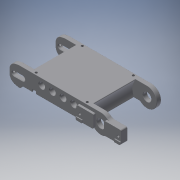
# Autodesk Inventor part: J007811
Saved by Autodesk Inventor 2018.3 (Build 223284000, 284)
## iProperties
Created: 2014-06-24
Material: VERO BLACK
Vendor: HHMI: JRC - ID&F
Document SubType Name: Modeling
Designer: ARNOLDJ
Density: 1.17 g/cm^3
Description: NRB MAIN BODY INSERTS
Mass: 114.449 g
Surface Area: 315.275 cm^2
Volume: 97.8198 cm^3
Appearance: Default
Project: COMMON
Part Number: J007811
RuleStatus: InUse
AfterDocSave0: file://Part Number Cleaner
LAB/DEPT: COMMON
REQUESTING SCIENTIST: COMMON
SURFACE ROUGHNESS: N/A
DESIGN DEPARTMENT: HHMI: JRC - ID&F
SPECIAL FINISH: NONE
ALTERED ITEM PART NUMBER: N/A
ALTERED ITEM VENDOR: N/A
ALTERED ITEM DESCRIPTION: N/A
Revision Number: 0
Autodesk Inventor part; units mm, degrees
sketch "Sketch1" plane through (0, 0, 0) normal (0, 0, 1) x (1, 0, 0)
  circle A0 centre (0, 0) radius 2.286
  circle A1 centre (98.552, 0) radius 4.7752
  line L0 (-5.7162, 13.208) -> (130.4794, 13.208) construction
  line L1 (0, 11.708) -> (98.552, 11.708)
  arc A2 (90.2495, -8.255) -> (98.552, 11.708) centre (98.552, 0) ccw
  line L2 (5.358, -8.255) -> (90.2495, -8.255)
  line L3 (0, 0) -> (0, -11.708) construction
  line L4 (0, -11.708) -> (-26.2981, -11.708) construction
  circle A3 centre (98.552, 0) radius 13.208 construction
  arc A4 (-3.81, 11.708) -> (-3.81, -11.708) centre (-3.81, 0) ccw
  line L5 (-3.81, -11.708) -> (1.905, -11.708)
  line L6 (-3.81, 11.708) -> (0, 11.708)
  circle A5 centre (98.552, 0) radius 11.708 construction
  line L7 (1.905, -11.708) -> (5.358, -8.255)
  circle A6 centre (-3.81, 0) radius 17.399 construction
  line L8 (-10.795, 9.3961) -> (-10.795, -9.3961)
  line L9 (0, 11.708) -> (-10.795, 9.3961)
  line L10 (-10.795, -9.3961) -> (0, -11.708)
  dimension "d233" = 23.416
  dimension "BRG_CLEAR" = 4.572
  dimension "d1" = 9.5504
  dimension "AXEL_CENTER" = 98.552
  dimension "TOP_CHAIN" = 13.208
  dimension "BELT_THICKNESS" = 1.5
  dimension "d111" = 3.81
  dimension "d226" = 11.708
  dimension "d232" = 8.255
  dimension "d235" = 135
  dimension "d236" = 1.905
  dimension "d237" = 26.416
  dimension "d238" = 34.798
  dimension "d335" = 10.795
  constraints: 22 end point, 6 centre point, 6 coincident, 6 point on circle, 5 horizontal, 4 tangent, 2 point on line, 2 vertical, 1 equal radius, 1 horizontal alignment, 1 parallel, 3 other
  measures "BRG_CLEAR" diameter of A0
  measures "d1" diameter of A1
  measures "AXEL_CENTER" distance of A1.centre point (0, 0)
  measures "TOP_CHAIN" distance from line of L0 point (0, 0)
  measures "BELT_THICKNESS" distance between parallel lines of L1 L0
  measures "d111" distance of point (0, 0) A4.centre
  measures "d226" distance from line of L1 point (0, 0)
  measures "d232" distance from line of L2 A1.centre
  measures "d235" angle of L2 L7
  measures "d236" horizontal distance of point (0, 0) L5.end
  measures "d237" diameter of A3
  measures "d238" diameter of A6
  measures "d335" distance from line of point (0, 0) L8
extrude "Extrusion1" add sketch "Sketch1" along normal mid plane 60.198 contours L1 A2 L2 L7 L5 L10 L8 L9
ref_plane "Work Plane1" through (0, 0, 6.5) normal (0, 0, 1) x (1, 0, 0)
sketch "Sketch2" plane through (0, 0, 6.5) normal (0, 0, 1) x (1, 0, 0)
  circle A0 centre (98.552, 0) radius 4.7752 projected
  circle A1 centre (0, 0) radius 2.286 projected
  line L0 (98.552, 11.708) -> (0, 11.708) projected
  arc A2 (90.2495, -8.255) -> (98.552, 11.708) centre (98.552, 0) ccw projected
  line L1 (5.358, -8.255) -> (90.2495, -8.255) projected
  line L2 (0, -11.708) -> (1.905, -11.708) projected
  line L3 (1.905, -11.708) -> (5.358, -8.255) projected
  line L4 (-10.795, 9.3961) -> (-10.795, -9.3961) projected
  line L5 (0, 11.708) -> (-10.795, 9.3961) projected
  line L6 (-10.795, -9.3961) -> (0, -11.708) projected
sketch "Sketch14" plane through (0, 0, 0) normal (0, 0, 1) x (1, 0, 0)
  point P0 (0, 0)
sketch "Sketch15" plane through (0, 0, 0) normal (0, 0, 1) x (1, 0, 0)
  line L0 (0, 11.708) -> (98.552, 11.708) projected
  circle A0 centre (98.552, 0) radius 4.7752 projected
  line L1 (90.2495, -8.255) -> (5.358, -8.255) projected
  circle A1 centre (98.552, 0) radius 17.4625
  circle A2 centre (0, 0) radius 2.286 projected
  circle A3 centre (0, 0) radius 17.4625
  circle A4 centre (-3.81, 0) radius 17.4625
  line L2 (-3.81, 17.4625) -> (0, 17.4625)
  dimension "d241" = 34.925
  dimension "d242" = 34.925
  dimension "d239" = 34.925
  constraints: 2 coincident, 2 end point, 2 horizontal, 2 vertical alignment, 1 centre point, 4 other
  measures "d239" diameter of A1
extrude "Extrusion6" cut sketch "Sketch15" along normal mid plane 50.038 contours A4 A3 L0 | L0 A3 L1 A4 | A4 A3 | A3 A4 | A1 | L1 A3 A4
fillet "Fillet13" radius 0.635 4 edges at (85.5959, 11.708, 0) (83.1639, -8.255, 0) (12.9561, 11.708, 0) (15.3881, -8.255, 0)
sketch "Sketch17" plane through (0, 0, 0) normal (0, 1, 0) x (-1, 0, 0)
  line L0 (-151.1165, 0) -> (65.8274, 0) projected
  line L1 (-118.2232, 10.8) -> (28.7239, 10.8) construction
  line L2 (-120.1245, -10.8) -> (34.8354, -10.8) construction
  point P0 (0, 0)
  dimension "d89" = 10.8
  dimension "d90" = 10.8
  constraints: 4 end point, 2 horizontal
  measures "d89" distance between parallel lines of L0 L1
  measures "d90" distance between parallel lines of L0 L2
sketch "Sketch18" plane through (0, 0, 0) normal (1, 0, 0) x (0, 1, 0)
  line L0 (-19.3771, 6.985) -> (16.5156, 6.985) construction
  line L1 (-20.38, -6.985) -> (18.235, -6.985) construction
  line L2 (-28.1031, 0) -> (25.958, 0) construction
  line L3 (0, 35.0266) -> (0, -35.0266) construction
  line L4 (11.708, 7.62) -> (11.073, 7.62)
  line L5 (11.073, 7.62) -> (11.073, 6.35)
  line L6 (11.073, 6.35) -> (11.708, 6.35)
  line L7 (11.708, 6.35) -> (11.708, 7.62)
  line L8 (11.708, -6.35) -> (11.073, -6.35)
  line L9 (11.073, -6.35) -> (11.073, -7.62)
  line L10 (11.073, -7.62) -> (11.708, -7.62)
  line L11 (11.708, -7.62) -> (11.708, -6.35)
  line L12 (11.708, 25.019) -> (11.708, -25.019) projected
  point P0 (0, 0)
  dimension "d94" = 0.635
  dimension "d243" = 0
  dimension "d244" = 0
  dimension "d367" = 12.7
  dimension "d368" = 1.27
  constraints: 20 end point, 4 horizontal, 4 parallel, 2 equal length, 2 perpendicular, 2 other
  measures "d94" distance of L4.start L4.end
  measures "d243" distance between parallel lines of L11 L12
  measures "d244" distance between parallel lines of L7 L12
  measures "d367" distance between parallel lines of L8 L6
  measures "d368" distance of L4.end L5.end
extrude "Extrusion8" [suppressed]
sketch "Sketch19" plane through (0, 0, 0) normal (0, 0, 1) x (1, 0, 0)
  line L0 (0, 0) -> (0, 6.4329) construction
  circle A0 centre (-5.08, 0) radius 2.413
  circle A1 centre (5.08, 0) radius 2.413
  line L1 (5.08, 0) -> (5.08, 2.413) construction
  line L2 (-5.08, 0) -> (-5.08, 2.413) construction
  line L3 (-5.08, 0) -> (-5.08, -2.413) construction
  line L4 (5.08, 0) -> (5.08, -2.413) construction
  line L5 (-5.08, 2.413) -> (5.08, 2.413)
  line L6 (-5.08, -2.413) -> (5.08, -2.413)
  arc A2 (0, 8.9) -> (3.6068, -8.1364) centre (0, 0) ccw construction
  dimension "d105" = 4.826
  dimension "d106" = 5.08
  dimension "d107" = 10.16
  constraints: 14 end point, 5 vertical, 4 point on circle, 4 tangent, 2 centre point, 2 horizontal, 1 equal radius
  measures "d105" diameter of A0
  measures "d106" distance of L2.start L0.start
  measures "d107" distance of L1.start L2.start
extrude "Extrusion9" cut sketch "Sketch19" along normal mid plane 88.9
mirror "Mirror4" about plane through (0, 0, 0) normal (0, 0, 1)
ref_plane "Work Plane3" through (0, 0, -28.5496) normal (0, 0, 1) x (1, 0, 0)
ref_plane "Work Plane5" through (-19.05, 0, 0) normal (1, 0, 0) x (0, 1, 0)
sketch "Sketch31" plane through (-19.05, 0, 0) normal (1, 0, 0) x (0, 1, 0)
  line L0 (9.3961, -30.099) -> (-9.3961, -30.099) projected
  line L1 (-9.3961, 30.099) -> (9.3961, 30.099) projected
  line L2 (-9.3961, -25.019) -> (9.3961, -25.019) projected
  line L3 (9.3961, 25.019) -> (-9.3961, 25.019) projected
  line L4 (0, 42.1386) -> (0, -42.1386) projected
  point P0 (0, 0)
  point P1 (0, -27.559)
  point P2 (0, 27.559)
  dimension "d338" = 5.08
  dimension "d339" = 2.54
  dimension "d403" = 0
  dimension "d404" = 2.54
  constraints: 1 vertical alignment
  measures "d338" distance between parallel lines of L0 L2
  measures "d339" distance from line of point (0, -27.559) L0
  measures "d403" distance from line of L4 point (0, -27.559)
  measures "d404" distance from line of point (0, 27.559) L3
hole "Hole6" at (-19.05, 0, -27.559) at (-19.05, 0, 27.559) direction (1, 0, 0) diameter 2.3622 depth 19.05 tip angle 118
ref_plane "Work Plane6" through (0, 0, 12.5095) normal (0, 0, 1) x (1, 0, 0)
ref_plane "Work Plane7" through (0, 0, 25.019) normal (0, 0, 1) x (1, 0, 0)
hole "Hole7" at (98.552, 0, 25.019) direction (0, 0, 1) diameter 9.5758 depth 25.4 tip angle 118
ref_plane "Work Plane9-Motor Drive Plane" through (135.1026, 0, 0) normal (1, 0, 0) x (0, 1, 0)
fillet "Fillet21" radius 2.54 5 edges at (1.905, -11.708, 27.559) (5.358, -8.255, 27.559) (1.905, -11.708, -27.559) (5.358, -8.255, -27.559) (90.2495, -8.255, -27.559)
fillet "Fillet22" radius 8.89 6 edges at (-10.795, 9.3961, -27.559) (-10.795, -9.3961, 27.559) (-10.795, -9.3961, -27.559) (-10.795, 9.3961, 27.559) (0, 11.708, -27.559) (0, 11.708, 27.559)
sketch "Sketch40" plane through (0, 0, 25.019) normal (0, 0, 1) x (1, 0, 0)
  circle A0 centre (98.552, 0) radius 4.7879 projected
  line L0 (0.9413, 11.708) -> (98.552, 11.708) projected
  arc A1 (90.2495, -8.255) -> (98.552, 11.708) centre (98.552, 0) ccw projected
  line L1 (90.2495, -8.255) -> (6.4101, -8.255) projected
  line L2 (92.202, -7.62) -> (71.882, -7.62)
  line L3 (71.882, -7.62) -> (71.882, 7.62)
  line L4 (71.882, 7.62) -> (92.202, 7.62)
  line L5 (92.202, 7.62) -> (92.202, -7.62)
  line L6 (92.202, -7.62) -> (71.882, 7.62) construction
  line L7 (71.882, -7.62) -> (92.202, 7.62) construction
  line L8 (104.902, -7.62) -> (125.222, -7.62)
  line L9 (125.222, -7.62) -> (125.222, 7.62)
  line L10 (125.222, 7.62) -> (104.902, 7.62)
  line L11 (104.902, 7.62) -> (104.902, -7.62)
  line L12 (104.902, -7.62) -> (125.222, 7.62) construction
  line L13 (125.222, -7.62) -> (104.902, 7.62) construction
  point P0 (0, 0)
  point P1 (82.042, 0)
  point P2 (115.062, 0)
  point P3 (82.042, 0)
  point P4 (115.062, 0)
  dimension "d343" = 6.35
  dimension "d344" = 6.35
  dimension "d345" = 26.67
  dimension "d346" = 26.67
  dimension "d347" = 15.24
  dimension "d348" = 15.24
  constraints: 24 end point, 6 midpoint, 4 parallel, 2 horizontal, 2 horizontal alignment, 2 perpendicular
  measures "d343" distance from line of L5 A0.centre
  measures "d344" distance from line of L11 A0.centre
  measures "d345" distance from line of A1.centre L3
  measures "d346" distance from line of L9 A0.centre
  measures "d347" distance of L2.end L3.end
  measures "d348" distance of L8.end L9.end
extrude "Extrusion22" add sketch "Sketch40" along normal blind 7.62 contours L8 L11 L10 A1 | A1 L10 L9 L8 | L2 L3 L4 L5
sketch "Sketch41" plane through (0, 0, 32.639) normal (0, 0, 1) x (1, 0, 0)
  circle A0 centre (98.552, 0) radius 4.7879 projected
  circle A1 centre (98.552, 0) radius 23 construction
  line L0 (71.882, -7.62) -> (79.502, -7.62)
  line L1 (79.502, -7.62) -> (79.502, -4.2418)
  line L2 (79.502, -4.2418) -> (71.882, -4.2418)
  line L3 (71.882, -4.2418) -> (71.882, -7.62)
  line L4 (125.222, -7.62) -> (117.602, -7.62)
  line L5 (117.602, -7.62) -> (117.602, -4.2418)
  line L6 (117.602, -4.2418) -> (125.222, -4.2418)
  line L7 (125.222, -4.2418) -> (125.222, -7.62)
  point P0 (0, 0)
  point P1 (75.552, 0)
  point P2 (121.552, 0)
  dimension "d351" = 46
  dimension "d359" = 7.62
  dimension "d360" = 7.62
  dimension "d361" = 4.2418
  constraints: 16 end point, 4 parallel, 2 horizontal, 2 perpendicular, 2 point on circle, 1 centre point, 1 coincident, 1 horizontal alignment, 1 point on line
  measures "d351" diameter of A1
  measures "d359" distance of L1.end L2.end
  measures "d360" distance of L5.end L6.end
  measures "d361" distance from line of L2 A1.start
hole "Hole8" at (75.552, 0, 32.639) at (121.552, 0, 32.639) direction (0, 0, -1) diameter 2.8956 depth 20.32 tip angle 118 clearance for "Socket Head Cap Screw" size "M2.5" standard "Ansi Metric M Profile"
ref_plane "Work Plane10" through (0, 0, 42.164) normal (0, 0, 1) x (1, 0, 0)
sketch "Sketch5" plane through (0, 0, 42.164) normal (0, 0, 1) x (1, 0, 0)
  circle A0 centre (97.79, 0) radius 4.7879
  circle A1 centre (-9.5263, 0.1013) radius 2.286
  line L0 (-75.7985, 4.088) -> (143.5735, 4.088)
  line L1 (0, 18.1055) -> (0, -20.875) projected
  line L2 (0.9413, 11.708) -> (98.552, 11.708) projected
  point P0 (27.94, 4.088)
  point P1 (53.34, 4.088)
  point P2 (40.64, 4.088)
  point P3 (66.04, 4.088)
  dimension "d33" = 25.4
  dimension "d34" = 12.7
  dimension "d405" = 40.64
  dimension "d406" = 7.62
  dimension "d407" = 3.9867
  dimension "d408" = 12.7
  constraints: 4 point on line, 2 centre point, 2 end point, 2 horizontal alignment
  measures "d33" distance of point (53.34, 4.088) point (27.94, 4.088)
  measures "d34" distance of point (53.34, 4.088) point (40.64, 4.088)
  measures "d405" distance from line of point (40.64, 4.088) L1
  measures "d406" distance from line of point (27.94, 4.088) L2
  measures "d407" vertical distance of point (27.94, 4.088) A1.centre
  measures "d408" distance of point (66.04, 4.088) point (53.34, 4.088)
hole "Hole2" at (27.94, 4.088, 42.164) at (53.34, 4.088, 42.164) at (40.64, 4.088, 42.164) at (66.04, 4.088, 42.164) direction (0, 0, -1) diameter 6.731 end through all
extrude "Extrusion23" add sketch "Sketch41" along normal blind 1.016 contours L3 L2 L1 L0 | L4 L5 L6 L7
fillet "Fillet23" radius 1.524 8 edges at (71.882, 7.62, 31.369) (92.202, 7.62, 31.369) (92.202, -7.62, 31.369) (104.902, 7.62, 31.369) (125.222, 7.62, 28.829) (125.222, -7.62, 29.337) (104.902, -7.62, 31.369) (71.882, -7.62, 31.877)
chamfer "Chamfer12" distance 0.381 angle 45 4 edges at (93.7768, 0, -30.099) (98.552, -4.7879, 30.099) (98.552, -4.7879, 25.019) (93.7768, 0, -25.019)
fillet "Fillet24" radius 6.35 2 edges at (107.4409, 7.62, 27.559) (107.4409, -7.62, 27.559)
fillet "Fillet25" radius 0.635 6 edges at (79.502, -4.2418, 33.147) (79.502, -7.62, 33.147) (71.882, -4.2418, 33.147) (117.602, -4.2418, 33.147) (125.222, -4.2418, 33.147) (117.602, -7.62, 33.147)
sketch "Sketch46" plane through (0, 0, 0) normal (0, 0, 1) x (1, 0, 0)
  circle A0 centre (27.94, 4.088) radius 3.3655 projected
  line L0 (22.352, 9.676) -> (33.528, 9.676)
  line L1 (33.528, 9.676) -> (33.528, -1.5)
  line L2 (33.528, -1.5) -> (22.352, -1.5)
  line L3 (22.352, -1.5) -> (22.352, 9.676)
  line L4 (22.352, 9.676) -> (33.528, -1.5) construction
  line L5 (33.528, 9.676) -> (22.352, -1.5) construction
  point P0 (0, 0)
  dimension "d409" = 11.176
  dimension "d410" = 11.176
  constraints: 12 end point, 2 midpoint, 2 parallel, 1 horizontal, 1 perpendicular
  measures "d409" distance of L1.end L2.end
  measures "d410" distance of L0.end L1.end
extrude "Extrusion26" cut sketch "Sketch46" along normal mid plane 48.26 contours A0 | L0 L1 L2 L3
pattern_linear "Rectangular Pattern2" count 4 spacing 12.7 along (1, 0, 0) of "Extrusion26"
sketch "Sketch42" plane through (90.2495, -8.255, 25.019) normal (0, -1, 0) x (1, 0, 0)
  line L0 (-90.2495, 21.3868) -> (-90.2495, -67.8688) projected
  line L1 (-157.0964, -25.019) -> (66.984, -25.019) projected
  line L2 (-13.0335, -42.799) -> (-68.9135, -42.799)
  line L3 (-68.9135, -42.799) -> (-68.9135, -7.239)
  line L4 (-68.9135, -7.239) -> (-13.0335, -7.239)
  line L5 (-13.0335, -7.239) -> (-13.0335, -42.799)
  line L6 (-13.0335, -42.799) -> (-68.9135, -7.239) construction
  line L7 (-68.9135, -42.799) -> (-13.0335, -7.239) construction
  line L8 (-76.4371, -50.038) -> (-76.4371, 0) projected
  line L9 (-5.5098, 0) -> (-5.5098, -50.038) projected
  point P0 (-90.2495, -25.019)
  point P1 (-40.9735, -25.019)
  dimension "d369" = 35.56
  dimension "d370" = 55.88
  dimension "d371" = 49.276
  dimension "d372" = 7.5236
  dimension "d373" = 7.5236
  constraints: 12 end point, 2 midpoint, 2 parallel, 1 horizontal, 1 perpendicular, 1 point on line
  measures "d369" distance of L2.end L3.end
  measures "d370" distance of L3.end L4.end
  measures "d371" distance from line of L0 point (-40.973, -25.019)
  measures "d372" distance between parallel lines of L8 L3
  measures "d373" distance between parallel lines of L5 L9
extrude "Extrusion24" cut sketch "Sketch42" against normal up to surface (17.931 mm away)
ref_plane "Work Plane11" through (50.8, 0, 0) normal (1, 0, 0) x (0, 1, 0)
sketch "Sketch44" plane through (98.552, 11.708, 30.099) normal (0, 1, 0) x (1, 0, 0)
  line L0 (-97.6107, 0) -> (0, 0) projected
  line L1 (-47.752, 72.9488) -> (-47.752, -16.3068) projected
  line L2 (-84.2374, 5.08) -> (-84.2374, 55.118) projected
  line L3 (-14.3146, 55.118) -> (-14.3146, 5.08) projected
  point P0 (-98.552, 30.099)
  point P1 (-79.756, 2.54)
  point P2 (-18.796, 2.54)
  point P3 (-49.276, 2.54)
  dimension "d389" = 32.004
  dimension "d390" = 28.956
  dimension "d391" = 2.54
  dimension "d399" = 30.48
  dimension "d400" = 4.4814
  dimension "d401" = 4.4814
  dimension "d402" = 2.54
  measures "d389" distance from line of L1 point (-79.756, 2.54)
  measures "d390" distance from line of L1 point (-18.796, 2.54)
  measures "d391" distance from line of L0 point (-79.756, 2.54)
  measures "d399" distance of point (-49.276, 2.54) point (-79.756, 2.54)
  measures "d400" distance from line of point (-79.756, 2.54) L2
  measures "d401" distance from line of L3 point (-18.796, 2.54)
  measures "d402" distance from line of point (-49.276, 2.54) L0
hole "Hole9" at (18.796, 11.708, 27.559) at (79.756, 11.708, 27.559) direction (0, -1, 0) diameter 2.794 end through all clearance for "Socket Head Cap Screw" size "M2.5" standard "Ansi Metric M Profile"
mirror "Mirror6" about plane through (0, 0, 0) normal (0, 0, 1) of "Hole9"
sketch "Sketch47" plane through (0, 0, 12.5095) normal (0, 0, 1) x (1, 0, 0)
  circle A0 centre (75.552, 0) radius 1.4478 projected
  line L0 (78.102, -1.4722) -> (75.552, -2.9445)
  line L1 (75.552, -2.9445) -> (73.002, -1.4722)
  line L2 (73.002, -1.4722) -> (73.002, 1.4722)
  line L3 (73.002, 1.4722) -> (75.552, 2.9445)
  line L4 (75.552, 2.9445) -> (78.102, 1.4722)
  line L5 (78.102, 1.4722) -> (78.102, -1.4722)
  line L6 (0, 18.1055) -> (0, -20.875) projected
  point P0 (0, 0)
  dimension "d416" = 5.1
  dimension "d417" = 0
  constraints: 12 end point, 1 coincident, 13 other
  measures "d416" distance between parallel lines of L5 L2
  measures "d417" angle of L2 L6
extrude "Extrusion27" cut sketch "Sketch47" along normal blind 7.62
fillet "Fillet28" radius 1.27 2 edges at (77.216, 1.9838, 15.1448) (77.216, -1.9838, 15.1448)
sketch "Sketch48" plane through (0, 0, 25.019) normal (0, 0, -1) x (-1, 0, 0)
  circle A0 centre (-121.552, 0) radius 1.4478 projected
  line L0 (-124.102, -1.4722) -> (-124.102, 1.4722)
  line L1 (-124.102, 1.4722) -> (-121.552, 2.9445)
  line L2 (-121.552, 2.9445) -> (-119.002, 1.4722)
  line L3 (-119.002, 1.4722) -> (-119.002, -1.4722)
  line L4 (-119.002, -1.4722) -> (-121.552, -2.9445)
  line L5 (-121.552, -2.9445) -> (-124.102, -1.4722)
  line L6 (0, -20.875) -> (0, 18.1055) projected
  point P0 (0, 0)
  dimension "d421" = 5.1
  dimension "d422" = 0
  constraints: 12 end point, 1 coincident, 13 other
  measures "d421" distance between parallel lines of L3 L0
  measures "d422" angle of L3 L6
extrude "Extrusion28" cut sketch "Sketch48" against normal blind 2.54
sketch "Sketch49" plane through (90.2495, -8.255, 25.019) normal (0, -1, 0) x (1, 0, 0)
  circle A0 centre (-71.4535, 2.54) radius 1.397 projected
  line L0 (-69.9812, 5.09) -> (-68.509, 2.54)
  line L1 (-68.509, 2.54) -> (-69.9812, -0.01)
  line L2 (-69.9812, -0.01) -> (-72.9257, -0.01)
  line L3 (-72.9257, -0.01) -> (-74.3979, 2.54)
  line L4 (-74.3979, 2.54) -> (-72.9257, 5.09)
  line L5 (-72.9257, 5.09) -> (-69.9812, 5.09)
  line L6 (-157.0964, -25.019) -> (66.984, -25.019) projected
  circle A1 centre (-10.4935, 2.54) radius 1.397 projected
  line L7 (-11.9657, -0.01) -> (-13.4379, 2.54)
  line L8 (-13.4379, 2.54) -> (-11.9657, 5.09)
  line L9 (-11.9657, 5.09) -> (-9.0212, 5.09)
  line L10 (-9.0212, 5.09) -> (-7.549, 2.54)
  line L11 (-7.549, 2.54) -> (-9.0212, -0.01)
  line L12 (-9.0212, -0.01) -> (-11.9657, -0.01)
  circle A2 centre (-71.4535, -52.578) radius 1.397 projected
  circle A3 centre (-10.4935, -52.578) radius 1.397 projected
  line L13 (-72.9257, -50.028) -> (-69.9812, -50.028)
  line L14 (-69.9812, -50.028) -> (-68.509, -52.578)
  line L15 (-68.509, -52.578) -> (-69.9812, -55.128)
  line L16 (-69.9812, -55.128) -> (-72.9257, -55.128)
  line L17 (-72.9257, -55.128) -> (-74.3979, -52.578)
  line L18 (-74.3979, -52.578) -> (-72.9257, -50.028)
  line L19 (-11.9657, -50.028) -> (-9.0212, -50.028)
  line L20 (-9.0212, -50.028) -> (-7.549, -52.578)
  line L21 (-7.549, -52.578) -> (-9.0212, -55.128)
  line L22 (-9.0212, -55.128) -> (-11.9657, -55.128)
  line L23 (-11.9657, -55.128) -> (-13.4379, -52.578)
  line L24 (-13.4379, -52.578) -> (-11.9657, -50.028)
  point P0 (-90.2495, -25.019)
  dimension "d425" = 5.1
  dimension "d426" = 0
  dimension "d427" = 5.1
  dimension "d428" = 5.1
  dimension "d429" = 5.1
  constraints: 48 end point, 4 coincident, 3 equal length, 52 other
  measures "d425" distance between parallel lines of L2 L5
  measures "d426" angle of L2 L6
  measures "d427" distance between parallel lines of L12 L9
  measures "d428" distance between parallel lines of L22 L19
  measures "d429" distance between parallel lines of L16 L13
extrude "Extrusion29" cut sketch "Sketch49" against normal blind 3
chamfer "Chamfer13" distance 0.635 angle 45 20 edges at (81.9673, -8.255, -28.829) (81.9644, -8.255, -26.284) (79.756, -8.255, -25.009) (77.5476, -8.255, -26.284) (77.5447, -8.255, -28.829) (21.0044, -8.255, -26.284) (18.796, -8.255, -25.009) (16.5876, -8.255, -26.284) (16.5847, -8.255, -28.829) (21.0073, -8.255, -28.829) (21.0073, -8.255, 28.829) (21.0044, -8.255, 26.284) (16.5876, -8.255, 26.284) (16.5847, -8.255, 28.829) (18.796, -8.255, 25.009) (81.9673, -8.255, 28.829) (81.9644, -8.255, 26.284) (79.756, -8.255, 25.009) (77.5476, -8.255, 26.284) (77.5447, -8.255, 28.829)
fillet "Fillet30" radius 0.635 6 edges at (81.234, -6.4375, -30.099) (78.278, -6.4375, -30.099) (20.274, -6.4375, -30.099) (17.318, -6.4375, -30.099) (20.274, -6.4375, 30.099) (17.318, -6.4375, 30.099)
chamfer "Chamfer14" distance 0.635 angle 45 11 edges at (74.277, 2.2084, 17.78) (76.7015, 2.2808, 17.78) (73.002, 0, 17.78) (74.277, -2.2084, 17.78) (76.7015, -2.2808, 17.78) (120.277, 2.2084, 25.019) (122.827, 2.2084, 25.019) (124.102, 0, 25.019) (122.827, -2.2084, 25.019) (120.277, -2.2084, 25.019) (119.002, 0, 25.019)
chamfer "Chamfer15" distance 0.635 angle 45 8 edges at (66.04, 7.4535, -30.099) (53.34, 7.4535, -30.099) (40.64, 7.4535, -30.099) (27.94, 7.4535, -30.099) (27.94, 7.4535, 30.099) (40.64, 7.4535, 30.099) (53.34, 7.4535, 30.099) (66.04, 7.4535, 30.099)
chamfer "Chamfer16" distance 0.635 angle 45 16 edges at (0, -2.413, -25.019) (-7.493, 0, -25.019) (0, 2.413, -25.019) (7.493, 0, -25.019) (0, -2.413, 30.099) (-7.493, 0, 30.099) (0, 2.413, 30.099) (7.493, 0, 30.099) (0, -2.413, 25.019) (7.493, 0, 25.019) (0, 2.413, 25.019) (-7.493, 0, 25.019) (0, -2.413, -30.099) (7.493, 0, -30.099) (0, 2.413, -30.099) (-7.493, 0, -30.099)
fillet "Fillet31" radius 0.381 77 edges at (0.0052, 11.6586, -25.019) (-2.3435, 11.2061, -25.019) (-8.8181, 7.7978, -25.019) (-10.795, 0, -25.019) (-8.8181, -7.7978, -25.019) (-1.8833, -11.3047, -25.019) (7.6279, 11.708, -25.019) (0.0052, 11.6586, -30.099) (-2.3435, 11.2061, -30.099) (-8.8181, 7.7978, -30.099) (-10.795, 0, -30.099) (-8.8181, -7.7978, -30.099) (-1.8833, -11.3047, -30.099) (109.5277, -4.0756, -30.099) (90.1371, -8.4139, -30.099) (85.7934, -8.255, -30.099) (82.1695, -8.255, -30.0774) (49.7466, 11.708, -30.099) (0.0052, 11.6586, 25.019) (-2.3435, 11.2061, 25.019) (-8.8181, 7.7978, 25.019) (-10.795, 0, 25.019) (-8.8181, -7.7978, 25.019) (-1.8833, -11.3047, 25.019) (7.6279, 11.708, 25.019) (102.491, 11.0255, 30.099) (107.8581, 7.9902, 30.099) (0.0052, 11.6586, 30.099) (-2.3435, 11.2061, 30.099) (-8.8181, 7.7978, 30.099) (-10.795, 0, 30.099) (-8.8181, -7.7978, 30.099) (-1.8833, -11.3047, 30.099) (49.7466, 11.708, 30.099) (109.5277, -4.0756, -25.019) (90.1371, -8.4139, -25.019) (85.6949, -8.255, -25.019) (91.3947, 11.708, -25.019) (102.491, 11.0255, 25.019) (107.8581, 7.9902, 25.019) (116.8462, 7.62, 25.019) (124.7756, 7.1736, 25.019) (125.222, 0, 25.019) (124.7756, -7.1736, 25.019) (116.8462, -7.62, 25.019) (107.8581, -7.9902, 25.019) (97.9551, -11.6928, 25.019) (91.3947, 11.708, 25.019) (5.4381, -8.4483, -25.019) (3.6315, -9.9815, -25.019) (1.8249, -11.5147, -25.019) (0.4264, -11.708, -25.019) (11.4126, -8.255, -25.019) (5.4381, -8.4483, 25.019) (3.6315, -9.9815, 25.019) (1.8249, -11.5147, 25.019) (0.4264, -11.708, 25.019) (11.4126, -8.255, 25.019) (77.3425, -8.255, -30.0774) (21.2095, -8.255, -30.0774) (49.276, -8.255, -30.099) (21.2095, -8.255, 30.0774) (49.4593, -8.255, 30.099) (16.3825, -8.255, -30.0774) (5.4381, -8.4483, -30.099) (3.6315, -9.9815, -30.099) (1.8249, -11.5147, -30.099) (0.4264, -11.708, -30.099) (11.3141, -8.255, -30.099) (5.4381, -8.4483, 30.099) (3.6315, -9.9815, 30.099) (1.8249, -11.5147, 30.099) (0.4264, -11.708, 30.099) (16.3825, -8.255, 30.0774) (11.3141, -8.255, 30.099) (107.8581, -7.9902, 30.099) (97.9551, -11.6928, 30.099)
chamfer "Chamfer17" distance 0.381 angle 45 25 edges at (71.628, 4.088, -17.78) (66.04, -1.5, -17.78) (60.452, 4.088, -17.78) (60.452, 4.088, -24.13) (53.34, -1.5, -17.78) (47.752, 4.088, -17.78) (46.228, 4.088, -17.78) (40.64, -1.5, -17.78) (35.052, 4.088, -17.78) (33.528, 4.088, -17.78) (27.94, -1.5, -17.78) (22.352, 4.088, -17.78) (58.928, 4.088, -17.78) (71.628, 4.088, 17.78) (66.04, -1.5, 17.78) (60.452, 4.088, 17.78) (58.928, 4.088, 17.78) (53.34, -1.5, 17.78) (47.752, 4.088, 17.78) (46.228, 4.088, 17.78) (40.64, -1.5, 17.78) (35.052, 4.088, 17.78) (33.528, 4.088, 17.78) (27.94, -1.5, 17.78) (22.352, 4.088, 17.78)
ref_plane "Work Plane2" through (0, 0, 0) normal (0, 0, 1) x (1, 0, 0)
ref_plane "Work Plane8-Driven Axis Plane" through (98.552, 0, 0) normal (1, 0, 0) x (0, 1, 0)
ref_plane "Work Plane12" through (0, 0, 0) normal (0, 0, 1) x (1, 0, 0)
equation "\"d34\" = 0.5 * d33"
body "Solid1"
